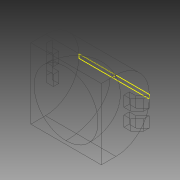
# Autodesk Inventor part: top
Saved by Autodesk Inventor 2014 SP2 (Build 180246200, 246)
## iProperties
Created: 2014-11-27
Part Number: top
Material: Generic
Document SubType Name: Modeling
Designer: No
Density: 1 g/cm^3
Appearance: Default
Mass: 53.4939 g
Surface Area: 158.315 cm^2
Volume: 53.4939 cm^3
Author: No
Autodesk Inventor part; units mm, degrees
ref_plane "XZ Plane" through (0, 0, 0) normal (0, 1, 0) x (-1, 0, 0)
sketch "Sketch1" plane through (0, 0, 0) normal (0, 1, 0) x (-1, 0, 0)
  line L0 (-26.5, 26.5) -> (26.5, 26.5)
  line L1 (26.5, 26.5) -> (26.5, -26.5)
  line L2 (26.5, -26.5) -> (-26.5, -26.5)
  line L3 (-26.5, -26.5) -> (-26.5, 26.5)
  line L4 (-26.5, 26.5) -> (26.5, -26.5) construction
  line L5 (26.5, 26.5) -> (-26.5, -26.5) construction
  point P0 (0, 0)
  dimension "d0" = 53
  dimension "d1" = 53
  constraints: 12 end point, 2 midpoint, 2 parallel, 1 horizontal, 1 perpendicular
  measures "d0" distance of L1.end L2.end
  measures "d1" distance of L0.end L1.end
extrude "Extrusion1" add sketch "Sketch1" along normal blind 36
sketch "Sketch2" plane through (0, 0, 0) normal (1, 0, 0) x (0, 1, 0)
  line L0 (0, 0) -> (33, 0) construction
  ellipse E0 centre (0, 0) end of major axis (33, 0) minor radius 24 (-33, 0) -> (33, 0) ccw
  line L1 (-33, 0) -> (33, 0)
  line L2 (46.2, 0) -> (-46.2, 0) projected
  dimension "d6" = 24
  dimension "d5" = 33
  constraints: 4 end point, 3 horizontal, 1 coincident, 4 other
  measures "d5" distance of L0.start L0.end
revolve "Revolution1" cut sketch "Sketch2" angle 360 about axis through (0, 0, 0) along (0, -1, 0)
sketch "Sketch3" plane through (26.5, 0, 26.5) normal (1, 0, 0) x (0, 0, -1)
  line L0 (0, 0) -> (0, 36) projected
  line L1 (29, 59.7326) -> (29, -35.1874)
  line L2 (16, 21) -> (24, 21)
  line L3 (24, 21) -> (24, 17)
  line L4 (24, 17) -> (16, 17)
  line L5 (16, 17) -> (16, 21)
  line L6 (16, 21) -> (24, 17) construction
  line L7 (24, 21) -> (16, 17) construction
  line L8 (0, 36) -> (53, 36) projected
  point P0 (26.5, 0)
  point P1 (20, 19)
  dimension "d8" = 8
  dimension "d9" = 4
  dimension "d10" = 10
  dimension "d14" = 15
  constraints: 14 end point, 3 parallel, 2 midpoint, 1 horizontal, 1 perpendicular, 1 vertical
  measures "d8" distance of L3.end L4.end
  measures "d9" distance of L2.end L3.end
  measures "d10" diameter of L3 L1
  measures "d14" distance between parallel lines of L8 L2
extrude "Extrusion2" add sketch "Sketch3" along normal blind 5
sketch "Sketch6" plane through (26.5, 17, 10.5) normal (0, 0, 1) x (1, 0, 0)
  line L0 (5, 4) -> (5, 0) projected
  line L1 (0, -17) -> (-53, -17) projected
  line L2 (0, -17) -> (0, 19) projected
  line L3 (-53, 19) -> (0, 19) projected
  line L4 (-53, -17) -> (-53, 19) projected
  line L5 (5, 4) -> (10, 9)
  line L6 (5, 4) -> (12.0711, 4) construction
  line L7 (10, 9) -> (10, 5)
  line L8 (10, 5) -> (5, 0)
  point P0 (-26.5, -17)
  dimension "d18" = 45
  dimension "d19" = 4
  constraints: 8 end point, 1 equal length, 1 horizontal, 1 perpendicular
  measures "d18" angle of L6 L5
  measures "d19" distance of L5.end L7.end
extrude "Extrusion3" add sketch "Sketch6" against normal up to surface (8 mm away) contours L5 L7 L8 L0
mirror "Mirror1" about plane through (0, 0, 0) normal (0, 0, 1) of "Extrusion2", "Extrusion3"
mirror "Mirror2" about plane through (0, 0, 0) normal (1, 0, 0) of "Extrusion3", "Extrusion2", "Mirror1"
fillet "Fillet1" radius 25 2 edges at (0, 36, 26.5) (0, 36, -26.5)
sketch "Sketch7" plane through (0, 36, 0) normal (0, 1, 0) x (1, 0, 0)
  line L0 (-26.5, 1.5) -> (26.5, 1.5) projected
  line L1 (-26.5, 1.5) -> (-26.5, -1.5) projected
  line L2 (26.5, -1.5) -> (-26.5, -1.5) projected
  line L3 (26.5, -1.5) -> (26.5, 1.5) projected
  point P0 (0, 0)
  point P1 (0, 0)
  constraints: 1 coincident
equation "\"d1\" = d0"
equation "\"d19\" = d9"
body "Solid1"
